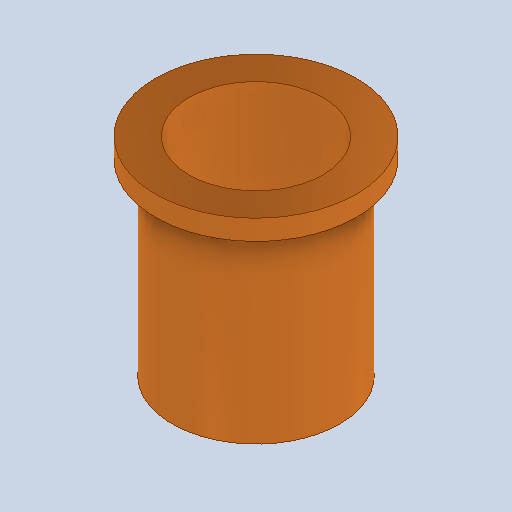
# Autodesk Inventor part: PlateSpacers
Saved by Autodesk Inventor 2023.2 (Build 272271030, 271C)
## iProperties
Created: 2023-03-23
Part Number: PlateSpacers
Material: Gold
Document SubType Name: Modeling
Designer: Luis Valente
Density: 19.3 g/cm^3
Appearance: Metal 1600F Hot
Author: Luis Valente
Autodesk Inventor part; units mm, degrees
ref_plane "YZ Plane" through (0, 0, 0) normal (1, 0, 0) x (0, 1, 0)
ref_plane "XZ Plane" through (0, 0, 0) normal (0, 1, 0) x (-1, 0, 0)
ref_plane "XY Plane" through (0, 0, 0) normal (0, 0, 1) x (1, 0, 0)
sketch "Sketch1" plane through (0, 0, 0) normal (0, 0, 1) x (1, 0, 0)
  line L0 (0, 0) -> (15, 0)
  line L1 (15, 0) -> (15, -3)
  line L2 (15, -3) -> (0, -3)
  line L3 (0, -3) -> (0, 0)
  dimension "d0" = 15
  dimension "d1" = 3
  constraints: 8 end point, 2 parallel, 1 horizontal, 1 perpendicular
  measures "d0" distance of L1.end L2.end
  measures "d1" distance of L0.end L1.end
revolve "Revolution1" add sketch "Sketch1" angle 360 about axis through (0, -3, 0) along (0, 1, 0)
sketch "Sketch2" plane through (0, 0, 0) normal (1, 0, 0) x (0, 1, 0)
  line L0 (-3, -15) -> (-3, 15) projected
  line L1 (-3, 0) -> (-31, 0)
  line L2 (-31, 0) -> (-31, -12.5)
  line L3 (-31, -12.5) -> (-3, -12.5)
  line L4 (-3, -12.5) -> (-3, 0)
  point P0 (0, 0)
  point P1 (-3, -12.5)
  dimension "d3" = 28
  dimension "d4" = 12.5
  constraints: 8 end point, 2 parallel, 1 horizontal, 1 midpoint, 1 perpendicular
  measures "d3" distance of L3.end L2.end
  measures "d4" distance of L2.end L1.end
revolve "Revolution2" add sketch "Sketch2" angle 360 about axis through (0, -3, 0) along (0, -1, 0)
sketch "Sketch3" plane through (0, -31, 0) normal (0, -1, 0) x (1, 0, 0)
  circle A0 centre (0, 0) radius 10
  dimension "d6" = 20
  constraints: 1 centre point, 1 coincident
  measures "d6" diameter of A0
extrude "Extrusion1" cut sketch "Sketch3" against normal blind 31
body "Solid1"
